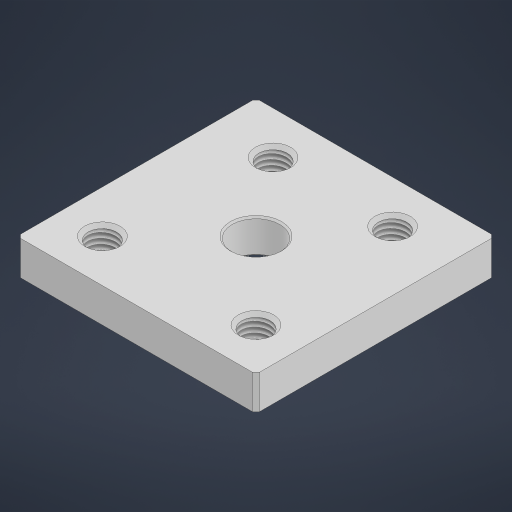
# Autodesk Inventor part: AP1-001
Saved by Autodesk Inventor 2024.3 (Build 283343000, 343)
## iProperties
Created: 2024-05-02
Part Number: AP1-001
Material: Generic
Document SubType Name: Modeling
Designer: fablabadmin
Density: 1 g/cm^3
Appearance: Default
Description: Plate bottom
Author: fablabadmin
Autodesk Inventor part; units mm, degrees
ref_plane "YZ Plane" through (0, 0, 0) normal (1, 0, 0) x (0, 1, 0)
ref_plane "XZ Plane" through (0, 0, 0) normal (0, 1, 0) x (-1, 0, 0)
ref_plane "XY Plane" through (0, 0, 0) normal (0, 0, 1) x (1, 0, 0)
sketch "Sketch1" plane through (0, 0, 0) normal (0, 1, 0) x (-1, 0, 0)
  line L0 (-35, 35) -> (35, 35)
  line L1 (35, 35) -> (35, -35)
  line L2 (35, -35) -> (-35, -35)
  line L3 (-35, -35) -> (-35, 35)
  line L4 (-35, 35) -> (35, -35) construction
  line L5 (35, 35) -> (-35, -35) construction
  line L6 (-22.5, 22.5) -> (22.5, 22.5) construction
  line L7 (22.5, 22.5) -> (22.5, -22.5) construction
  line L8 (22.5, -22.5) -> (-22.5, -22.5) construction
  line L9 (-22.5, -22.5) -> (-22.5, 22.5) construction
  line L10 (-22.5, 22.5) -> (22.5, -22.5) construction
  line L11 (22.5, 22.5) -> (-22.5, -22.5) construction
  circle A0 centre (0, 0) radius 7
  line L12 (17.5, 22.5) -> (-17.5, 22.5) construction
  line L13 (-17.5, 22.5) -> (-17.5, -22.5) construction
  line L14 (-17.5, -22.5) -> (17.5, -22.5) construction
  line L15 (17.5, -22.5) -> (17.5, 22.5) construction
  line L16 (49, 0) -> (-49, 0) construction
  line L17 (0, -49) -> (0, 49) construction
  dimension "d0" = 70
  dimension "d1" = 45
  dimension "d2" = 14
  dimension "d19" = 70
  dimension "d20" = 35
  dimension "d21" = 45
  dimension "d25" = 12.5
  dimension "d26" = 17.5
  constraints: 32 end point, 6 parallel, 5 coincident, 4 midpoint, 3 horizontal, 3 perpendicular, 3 point on line, 1 centre point, 1 other
  measures "d0" distance of L1.end L2.end
  measures "d1" distance of L7.end L8.end
  measures "d2" diameter of A0
  measures "d19" distance of L2.end L0.start
  measures "d20" distance of L13.end L14.end
  measures "d21" distance of L8.end L6.start
  measures "d25" distance between parallel lines of L7 L1
  measures "d26" distance between parallel lines of L1 L15
extrude "Extrusion1" add sketch "Sketch1" against normal blind 10
hole "Hole1" at (-22.5, 0, 22.5) at (22.5, 0, 22.5) at (-17.5, 0, -22.5) at (17.5, 0, -22.5) direction (0, -1, 0) diameter 8.376 end through all thread size "M10x1.5" class "6H" standard "ISO Metric profile"
chamfer "Chamfer1" distance 1 angle 45 8 edges at (-17.5, 0, -26.688) (17.5, 0, -26.688) (22.5, 0, 18.312) (-22.5, 0, 18.312) (-22.5, -10, 18.312) (-17.5, -10, -26.688) (17.5, -10, -26.688) (22.5, -10, 18.312)
chamfer "Chamfer2" distance 0.5 angle 45 2 edges at (7, 0, 0) (7, -10, 0)
chamfer "Chamfer3" distance 1 angle 45 4 edges at (-35, -5, 35) (-35, -5, -35) (35, -5, -35) (35, -5, 35)
body "Solid1"
